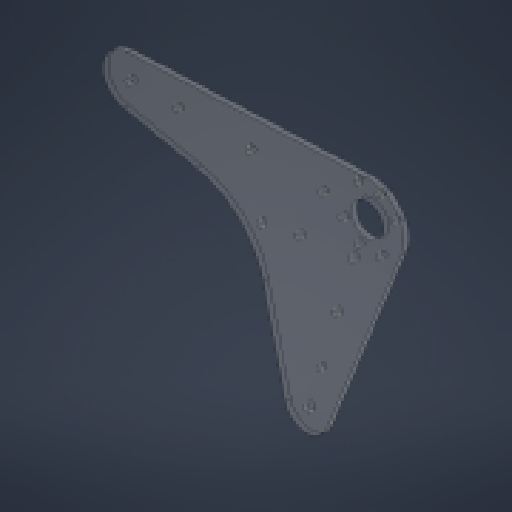
# Autodesk Inventor part: 4Bar_Input Side
Saved by Autodesk Inventor 2026.1 (Build 301233020, 233B)
## iProperties
Created: 2026-01-17
Part Number: 4Bar_Input Side
Material: Polycarbonate, Clear
Document SubType Name: Modeling
Designer: 110
Density: 1.2 g/cm^3
Appearance: Polycarbonate - Clear
Mass: 148.348 g
Surface Area: 573.548 cm^2
Volume: 123.623 cm^3
Author: 110
Autodesk Inventor part; units mm, degrees
ref_plane "YZ Plane" through (0, 0, 0) normal (1, 0, 0) x (0, 1, 0)
ref_plane "XZ Plane" through (0, 0, 0) normal (0, 1, 0) x (-1, 0, 0)
ref_plane "XY Plane" through (0, 0, 0) normal (0, 0, 1) x (1, 0, 0)
sketch "Sketch1" plane through (0, 0, 0) normal (0, 0, 1) x (1, 0, 0)
  arc A0 (-0.9706, 22.37) -> (-4.6554, -21.9018) centre (0, 0) ccw
  circle A1 centre (215.9, 0) radius 31.75 construction
  line L0 (-0.9706, 22.37) -> (214.5237, 31.7202)
  arc A2 (121.9186, -96.2694) -> (62.9615, -36.2742) centre (47.1186, -110.809) ccw
  line L1 (62.9615, -36.2742) -> (-4.6554, -21.9018)
  line L2 (121.9186, -96.2694) -> (136.3888, -170.7123)
  arc A3 (244.8834, -12.9625) -> (214.5237, 31.7202) centre (215.9, 0) ccw
  line L3 (244.8834, -12.9625) -> (172.4788, -174.8548)
  arc A4 (136.3888, -170.7123) -> (172.4788, -174.8548) centre (155.0888, -167.0773) ccw
  line L4 (0, 0) -> (203.2, 0) construction
  line L5 (215.9, 0) -> (155.0888, -167.0773) construction
  line L6 (0, 85.8367) -> (0, -233.7262) construction
  line L7 (-80.4559, 0) -> (313.641, 0) construction
  line L8 (0, 0) -> (215.9, 0) construction
  dimension "d30" = 63.5
  dimension "d31" = 44.7822
  dimension "d32" = 76.2
  dimension "d34" = 177.8
  dimension "d39" = 19.05
  dimension "d40" = 12
  dimension "d41" = 31
  dimension "d80" = 22.3911
  dimension "d86" = 215.9
  dimension "d87" = 0
  dimension "d101" = 70
  constraints: 15 end point, 10 point on circle, 8 tangent, 5 centre point, 4 coincident, 1 collinear, 1 concentric
  measures "d30" diameter of A1
  measures "d31" diameter of A0
  measures "d32" radius of A2
  measures "d34" distance of L5.start L5.end
  measures "d39" radius of A4
  measures "d40" angle of L1 L4
  measures "d41" angle of L2 L5
  measures "d80" radius of A0
  measures "d86" distance of L4.start L5.start
  measures "d87" distance between parallel lines of L8 L4
  measures "d101" angle of L4 L5
extrude "Extrusion1" add sketch "Sketch1" along normal blind 4.7625
sketch "Sketch2" plane through (0, 0, 4.7625) normal (0, 0, 1) x (1, 0, 0)
  arc A0 (136.3888, -170.7123) -> (172.4788, -174.8548) centre (155.0888, -167.0773) ccw projected
  line L0 (214.5237, 31.7202) -> (-0.9706, 22.37) projected
  arc A1 (-0.9706, 22.37) -> (-4.6554, -21.9018) centre (0, 0) ccw projected
  line L1 (-4.6554, -21.9018) -> (62.9615, -36.2742) projected
  arc A2 (121.9186, -96.2694) -> (62.9615, -36.2742) centre (47.1186, -110.809) ccw projected
  line L2 (121.9186, -96.2694) -> (136.3888, -170.7123) projected
  line L3 (172.4788, -174.8548) -> (244.8834, -12.9625) projected
  arc A3 (244.8834, -12.9625) -> (214.5237, 31.7202) centre (215.9, 0) ccw projected
  constraints: 1 coincident
hole "Structure Holes" at (155.0888, -167.0773, 4.7625) at (0, 0, 4.7625) direction (0, 0, -1) diameter 6.35 end through all
sketch "Sketch4" plane through (0, 0, 4.7625) normal (0, 0, 1) x (1, 0, 0)
  arc A0 (136.3888, -170.7123) -> (172.4788, -174.8548) centre (155.0888, -167.0773) ccw projected
  line L0 (214.5237, 31.7202) -> (-0.9706, 22.37) projected
  arc A1 (-0.9706, 22.37) -> (-4.6554, -21.9018) centre (0, 0) ccw projected
  line L1 (-4.6554, -21.9018) -> (62.9615, -36.2742) projected
  arc A2 (121.9186, -96.2694) -> (62.9615, -36.2742) centre (47.1186, -110.809) ccw projected
  line L2 (121.9186, -96.2694) -> (136.3888, -170.7123) projected
  line L3 (172.4788, -174.8548) -> (244.8834, -12.9625) projected
  arc A3 (244.8834, -12.9625) -> (214.5237, 31.7202) centre (215.9, 0) ccw projected
  line L4 (0, 0) -> (114.3, -50.8) construction
  dimension "d83" = 114.3
  dimension "d84" = 50.8
  constraints: 2 coincident, 2 end point
  measures "d83" horizontal distance of L4.start L4.end
  measures "d84" vertical distance of L4.start L4.end
hole "BearingHole" at (215.9, 0, 4.7625) direction (0, 0, -1) diameter 28.575 end through all
hole "Hole4" at (114.3, -50.8, 4.7625) direction (0, 0, -1) diameter 5.1054 end through all clearance for "Socket Head Cap Screw" size "#10" standard "Ansi Unified Screw Threads"
sketch "Sketch3" plane through (0, 0, 0) normal (0, 0, -1) x (-1, 0, 0)
  line L0 (0, 0) -> (-206.375, 0) construction
  circle A0 centre (-155.0888, -167.0773) radius 3.175 projected
  line L1 (-206.375, 0) -> (-155.0888, -167.0773) construction
  line L2 (-68.9435, 0) -> (-166.0461, -131.3812) construction
  line L3 (-117.4948, -65.6906) -> (-148.1345, -43.0451) construction
  point P0 (-215.9, 0)
  point P1 (-168.275, 0)
  point P2 (-104.775, 0)
  point P3 (-41.275, 0)
  point P4 (-195.1947, -36.4227)
  point P5 (-180.2876, -84.9862)
  point P6 (-165.3805, -133.5498)
  dimension "d10" = 137.4315
  dimension "d11" = 137.4315
  dimension "d12" = 38.1
  dimension "d43" = 38.1
  dimension "d46" = 63.5
  dimension "d51" = 38.1
  dimension "d54" = 50.8
  constraints: 8 end point, 4 point on line, 1 coincident, 1 horizontal, 1 horizontal alignment, 1 midpoint, 1 perpendicular, 5 other
  measures "d10" distance of L0.end L2.end
  measures "d11" distance of L0.end L2.start
  measures "d12" distance of L3.start L3.end
  measures "d43" distance of point (-168.275, 0) L0.end
  measures "d46" distance of point (-168.275, 0) point (-104.775, 0)
  measures "d51" distance of point (-195.195, -36.423) L0.end
  measures "d54" distance of point (-195.195, -36.423) point (-180.288, -84.986)
hole "Offset Holes" at (168.275, 0, 0) at (195.1947, -36.4227, 0) at (180.2876, -84.9862, 0) at (165.3805, -133.5498, 0) at (148.1345, -43.0451, 0) at (104.775, 0, 0) at (41.275, 0, 0) direction (0, 0, 1) diameter 5.1054 end through all clearance for "Flat Head Machine Screw (82)" size "#10" standard "Ansi Unified Screw Threads"
ref_plane "Inner Pitch Plane" through (0, 0, 0) normal (1, 0, 0) x (0, 1, 0)
sketch "Sketch6" plane through (0, 0, 4.7625) normal (0, 0, 1) x (1, 0, 0)
  arc A0 (244.8834, -12.9625) -> (214.5237, 31.7202) centre (215.9, 0) ccw projected
  line L0 (215.9, 0) -> (226.27, 23.1867) construction
  line L1 (172.4788, -174.8548) -> (244.8834, -12.9625) projected
  point P0 (0, 0)
  point P1 (206.8372, 23.7282)
  point P2 (192.7133, 10.37)
  point P3 (192.1718, -9.0628)
  point P4 (205.53, -23.1867)
  point P5 (224.9628, -23.7282)
  point P6 (239.0867, -10.37)
  point P7 (239.6282, 9.0628)
  dimension "d89" = 25.4
  dimension "d92" = 360
  constraints: 2 end point, 1 parallel, 9 other
  measures "d89" distance of L0.start L0.end
hole "Hole5" at (226.27, 23.1867, 4.7625) at (206.8372, 23.7282, 4.7625) at (192.1718, -9.0628, 4.7625) at (205.53, -23.1867, 4.7625) at (224.9628, -23.7282, 4.7625) at (239.6282, 9.0628, 4.7625) direction (0, 0, -1) diameter 4.9784 depth 13.6144 tip angle 118 clearance for "Flat Head Machine Screw (82)" size "#10" standard "Ansi Unified Screw Threads"
equation "\"d10\" = d11"
equation "\"d51\" = d43"
body "Solid1"
